wheel v35 (Autodesk Fusion 360 design; units mm, degrees)
Autodesk Fusion 360 part; units mm, degrees
sketch "スケッチ1" plane through (0, 0, 0) normal (0, 0, 1) x (1, 0, 0)
  circle A0 centre (0, 0) radius 5.4
  circle A1 centre (0, 0) radius 5
  circle A2 centre (0, 0) radius 1
  circle A3 centre (0, 0) radius 1.6
  line L0 (-0.2, 1.5875) -> (-0.2, 4.996)
  line L1 (0.2, 4.996) -> (0.2, 1.5875)
  line L2 (-1.2748, -0.9669) -> (-4.2267, -2.6712)
  line L3 (-4.4267, -2.3248) -> (-1.4748, -0.6205)
  line L4 (1.4748, -0.6205) -> (4.4267, -2.3248)
  line L5 (4.2267, -2.6712) -> (1.2748, -0.9669)
  circle A4 centre (0, 0) radius 4.6
  dimension "d1" = 10.8
  dimension "d2" = 10
  dimension "d3" = 2
  dimension "d4" = 3.2
  dimension "d5" = 0.4
  dimension "d7" = 360
  dimension "d17" = 9.2
  measures "d1" diameter of A0
  measures "d2" diameter of A1
  measures "d3" diameter of A2
  measures "d4" diameter of A3
  measures "d5" distance of L0 L1
  measures "d17" diameter of A4
extrude "押し出し1" add sketch "スケッチ1" along normal blind 3.5 contours A0 | A1 L0 L1 A4 | A1 L4 L5 A4 | A3 L0 L1 A4 | A3 L4 L5 A4 | A1 L2 L3 A4 | A3 L2 L3 A4
extrude "押し出し5" add sketch "スケッチ1" along normal blind 2 from surface at 2.5 contours A1 L1 L4 A4 | A1 L0 L1 A4 | A1 L4 L5 A4 | A1 L0 L3 A4 | A3 L0 L1 A4 | A1 L2 L5 A4 | A3 L4 L5 A4 | A1 L2 L3 A4 | A3 L2 L3 A4
extrude "押し出し2" add sketch "スケッチ1" along normal blind 6 contours A3
fillet "フィレット2" radius 0.2 6 edges at (-4.3301, 2.5, 2.5) (-3.9837, 2.3, 2.5) (3.9837, 2.3, 2.5) (4.3301, 2.5, 2.5) (0, -5, 2.5) (0, -4.6, 2.5)
fillet "フィレット2" radius 0.3 18 edges at (0.2, 4.5957, 3.5) (-0.2, 4.5957, 3.5) (1.2748, -0.9669, 2.25) (1.4748, -0.6205, 2.25) (-1.2748, -0.9669, 2.25) (0.2, 4.996, 1.25) (-0.2, 4.996, 1.25) (-1.4748, -0.6205, 2.25) (-0.2, 1.5875, 2.25) (0.2, 1.5875, 2.25) (4.0799, -2.1246, 3.5) (3.8799, -2.471, 3.5) (4.2267, -2.6712, 1.25) (4.4267, -2.3248, 1.25) (-4.0799, -2.1246, 3.5) (-3.8799, -2.471, 3.5) (-4.2267, -2.6712, 1.25) (-4.4267, -2.3248, 1.25)
